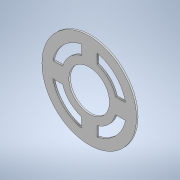
# Autodesk Inventor part: пп
Saved by Autodesk Inventor 2021 (Build 250183000, 183)
## iProperties
Created: 2024-03-30
Part Number: пп
Material: Типовые
Document SubType Name: Modeling
Designer: Мария
Density: 1 g/cm^3
Appearance: По умолчанию
Author: Мария
Autodesk Inventor part; units mm, degrees
ref_plane "YZ Plane" through (0, 0, 0) normal (1, 0, 0) x (0, 1, 0)
ref_plane "XZ Plane" through (0, 0, 0) normal (0, 1, 0) x (-1, 0, 0)
ref_plane "XY Plane" through (0, 0, 0) normal (0, 0, 1) x (1, 0, 0)
sketch "Эскиз1" plane through (0, 0, 0) normal (0, 0, 1) x (1, 0, 0)
  circle A0 centre (0, 0) radius 15
  circle A1 centre (0, 0) radius 6.45
  dimension "d0" = 12.9
  dimension "d1" = 30
  constraints: 2 centre point, 2 coincident
  measures "d0" diameter of A1
  measures "d1" diameter of A0
extrude "Выдавливание1" add sketch "Эскиз1" along normal blind 0.5
sketch "Эскиз2" plane through (0, 0, 0) normal (0, 0, 1) x (1, 0, 0)
  circle A0 centre (0, 0) radius 8.7833
  circle A1 centre (0, 0) radius 6.45 projected
  circle A2 centre (0, 0) radius 11.7833
  circle A3 centre (0, 0) radius 14.1167
  circle A4 centre (0, 0) radius 15
  circle A5 centre (0, 0) radius 15 construction
  line L0 (0, 0) -> (15, 0) construction
  line L1 (0, 0) -> (-15, 0) construction
  line L2 (0, 0) -> (0, -15) construction
  line L3 (11.5151, 2.5) -> (8.42, 2.5)
  line L4 (11.5151, -2.5) -> (8.42, -2.5)
  line L5 (0, 0) -> (-15, 0) construction
  line L6 (0, 0) -> (15, 0) construction
  line L7 (0, 0) -> (0, 15) construction
  arc A6 (8.42, 2.5) -> (0.5895, 8.7635) centre (0, 0) ccw
  arc A7 (11.5151, 2.5) -> (0.6972, 11.7627) centre (0, 0) ccw
  line L8 (0, 0) -> (10.6066, -10.6066) construction
  line L9 (9.6222, -10.3293) -> (10.2472, -10.9543)
  line L10 (10.3293, -9.6222) -> (10.9543, -10.2472)
  line L11 (2.5, -11.5151) -> (2.5, -8.42)
  line L12 (-2.5, -11.5151) -> (-2.5, -8.42)
  line L13 (-11.5151, -2.5) -> (-8.42, -2.5)
  line L14 (-11.5151, 2.5) -> (-8.42, 2.5)
  line L15 (-2.5, 11.5151) -> (-2.5, 8.42)
  line L16 (2.5, 11.5151) -> (2.5, 8.42)
  line L17 (9.6222, 10.3293) -> (10.2472, 10.9543)
  line L18 (10.3293, 9.6222) -> (10.9543, 10.2472)
  line L19 (-10.3293, 9.6222) -> (-10.9543, 10.2472)
  line L20 (-9.6222, 10.3293) -> (-10.2472, 10.9543)
  line L21 (-9.6222, -10.3293) -> (-10.2472, -10.9543)
  line L22 (-10.3293, -9.6222) -> (-10.9543, -10.2472)
  point P0 (2.5, -8.42)
  point P1 (2.5, -11.5151)
  point P2 (-8.42, -2.5)
  point P3 (-11.5151, -2.5)
  point P4 (-2.5, -11.5151)
  point P5 (-2.5, 8.42)
  point P6 (-2.5, 11.5151)
  point P7 (-11.5151, 2.5)
  point P8 (-8.42, 2.5)
  point P9 (2.5, 11.5151)
  point P10 (-10.2472, 10.9543)
  point P11 (-9.6222, 10.3293)
  point P12 (9.6222, 10.3293)
  point P13 (10.2472, 10.9543)
  point P14 (10.9543, 10.2472)
  point P15 (10.3293, 9.6222)
  point P16 (-10.9543, -10.2472)
  point P17 (-10.3293, -9.6222)
  point P18 (-10.9543, 10.2472)
  point P19 (-9.6222, -10.3293)
  point P20 (-10.2472, -10.9543)
  dimension "d4" = 2.3333
  dimension "d5" = 3
  dimension "d6" = 2.3333
  dimension "d7" = 0.8833
  dimension "d8" = 90
  dimension "d9" = 90
  dimension "d13" = 90
  dimension "d14" = 90
  dimension "d20" = 5
  dimension "d23" = 45
  dimension "d24" = 1
  dimension "d27" = 360
  dimension "d31" = 360
  dimension "d33" = 0.8833
  constraints: 46 end point, 14 point on circle, 6 centre point, 6 coincident, 2 parallel, 2 vertical, 60 other
  measures "d4" radial gap between concentric circles of A0 A1
  measures "d5" radial gap between concentric circles of A2 A0
  measures "d6" radial gap between concentric circles of A2 A3
  measures "d7" radial gap between concentric circles of A4 A3
  measures "d8" angle of L2 L1
  measures "d9" angle of L0 L2
  measures "d13" angle of L7 L5
  measures "d14" angle of L7 L6
  measures "d20" distance between parallel lines of L3 L4
  measures "d23" angle of L6 L8
  measures "d24" distance between parallel lines of L9 L10
extrude "Выдавливание2" cut sketch "Эскиз2" along normal through all contours A0 L16 A2 L3 | L4 A2 L11 A0 | L12 A2 L13 A0 | A0 L14 A2 L15
equation "\"d6\" = d4"
equation "\"d7\" = d33"
equation "\"d9\" = d8"
equation "\"d13\" = d8"
equation "\"d14\" = d8"
